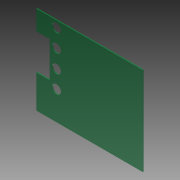
# Autodesk Inventor part: lcd_standoff
Saved by Autodesk Inventor 2014 (Build 180170000, 170)
## iProperties
Created: 2013-07-01
Part Number: lcd_standoff
Document SubType Name: Modeling
Designer: Administrator
Density: 1 g/cm^3
Material: Generic
Appearance: Clear - Green 1
Author: Administrator
Autodesk Inventor part; units mm, degrees
ref_plane "YZ Plane" through (0, 0, 0) normal (1, 0, 0) x (0, 1, 0)
ref_plane "XZ Plane" through (0, 0, 0) normal (0, 1, 0) x (-1, 0, 0)
ref_plane "XY Plane" through (0, 0, 0) normal (0, 0, 1) x (1, 0, 0)
sketch "Sketch1" plane through (0, 0, 0) normal (0, 0, 1) x (1, 0, 0)
  line L0 (4.5995, 3.2228) -> (80.3423, 3.2228)
  line L1 (80.3423, 3.2228) -> (80.3423, 65.9862)
  line L2 (80.3423, 65.9862) -> (4.5995, 65.9862)
  line L3 (4.5995, 65.9862) -> (4.5995, 3.2228)
  point P0 (0, 0)
  dimension "d0" = 75.7428
  dimension "d1" = 62.7634
  constraints: 8 end point
  measures "d0" distance of L1.end L2.end
  measures "d1" distance of L2.end L0.start
extrude "Extrusion1" add sketch "Sketch1" along normal blind 0.7937
sketch "Sketch4" plane through (0, 0, 0.7937) normal (0, 0, 1) x (1, 0, 0)
  line L0 (4.5995, 3.2228) -> (4.5995, 65.9862) projected
  line L1 (4.5995, 65.9862) -> (80.3423, 65.9862) projected
  line L2 (4.5995, 52.067) -> (14.2094, 52.067)
  line L3 (14.2094, 52.067) -> (14.2094, 26.667)
  line L4 (14.2094, 26.667) -> (4.5995, 26.667)
  line L5 (4.5995, 26.667) -> (4.5995, 52.067)
  point P0 (0, 0)
  dimension "d18" = 13.9192
  dimension "d19" = 25.4
  constraints: 8 end point, 2 parallel, 1 horizontal, 1 perpendicular, 1 point on line
  measures "d18" distance between parallel lines of L1 L2
  measures "d19" distance of L2.end L3.end
extrude "Extrusion4" cut sketch "Sketch4" against normal through all
sketch "Sketch5" plane through (0, 0, 0.7937) normal (0, 0, 1) x (1, 0, 0)
  line L0 (4.5995, 65.9862) -> (80.3423, 65.9862) projected
  line L1 (4.5995, 52.067) -> (4.5995, 65.9862) projected
  circle A0 centre (19.0208, 61.2935) radius 3.175
  circle A1 centre (19.0208, 48.7936) radius 3.175
  circle A2 centre (19.0208, 36.0437) radius 3.175
  circle A3 centre (19.0208, 23.5438) radius 3.175
  point P0 (0, 0)
  dimension "d20" = 6.35
  dimension "d21" = 14.4213
  dimension "d28" = 12.4999
  dimension "d29" = 12.7499
  dimension "d30" = 12.4999
  dimension "d31" = 4.6927
  constraints: 4 centre point, 3 equal radius, 3 vertical alignment
  measures "d20" diameter of A0
  measures "d21" distance from line of L1 A0.centre
  measures "d28" distance of A2.centre A3.centre
  measures "d29" distance of A1.centre A2.centre
  measures "d30" distance of A1.centre A0.centre
  measures "d31" distance from line of L0 A0.centre
extrude "Extrusion5" cut sketch "Sketch5" against normal through all
equation "\"d30\" = d28"
body "Solid1"
